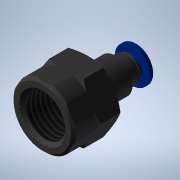
# Autodesk Inventor part: 190650 QSF-1/4-4-B
Saved by Autodesk Inventor 2021 (Build 250183000, 183)
## iProperties
Created: 2026-09-15
Part Number: 190650 QSF-1/4-4-B
Material: Generic
Catalog Web Link: www.3dfindit.com
Description: QSF-...-B-Push-in fitting
Vendor: FESTO
Document SubType Name: Modeling
Designer: psAdmin
Manufacturer: FESTO
Mass: 21 g
Surface Area: 21.8176 cm^2
Volume: 2.85568 cm^3
Density: 1 g/cm^3
Appearance: PSOLRGB-176-176-176
Category: PARTsolutions
Company: FESTO
Title: 190650 QSF-1/4-4-B
Author: Cadenas PARTsolutions
Comments: Push-in fitting
PSOL_IDENT_0: {$CADENAS_DATA/23d-libs/festo/parts/q/qsf/qsf_b.prj},179 {VTYP=3D},{NB=190650 QSF-1/4-4-B},{LINA=190
PSOL_IDENT_1: 650 QSF-1/4-4-B},{NN=QSF-...-B},{DATE=05.05.2026 15:29:25},{GEOMDATE=01.04.2025 10:00:39},{VERSION=}
PSOL_IDENT_2: ,{LINEID=40},{WBVAR=},{WBNUMERIC=}  {NB=190650 QSF-1/4-4-B},{LINA=190650 QSF-1/4-4-B},{KT=DUMMY},{TN
PSOL_IDENT_3: R=190650},{TYP=QSF-1/4-4-B},{D1=G1/4},{NENN=3.000},{D2=4},{D5=7.5},{L1=26.9},{L2=9},{SW=17},{T=14.9}
PSOL_IDENT_4: ,{CNSMASSEXACT=0.021},{D1N=13.157},{Z=9.9},{L3=20.600},{L3D1=17.600},{L3D2=9.700},{L4=7.000},{L5=7.6
PSOL_IDENT_5: 00},{GTIN=4052568042851},{REACH=Ja},{REACHSVHC=Ja},{REACHHAZSUBS=7439-92-1},{REACHSCIP=3732228b-b396
PSOL_IDENT_6: -49b9-8f0d-ee75d35d3f40},{REACHVALDATE=05.03.2025}
NB: 190650 QSF-1/4-4-B
NN: QSF-...-B
NT: Push-in fitting
NBSYN: $TNR. $TYP.
LINA: 190650 QSF-1/4-4-B
CATALOG: Festo
TNR: 190650
TYP: QSF-1/4-4-B
D1: G1/4
NENN: 3
D2: 4
D5: 7.5
L1: 26.9
L2: 9
SW: 17
T: 14.9
CNSMASSEXACT: 0.021
GTIN: 4052568042851
REACH: Yes
REACHSVHC: Yes
REACHHAZSUBS: 7439-92-1
REACHVALDATE: 05.03.2025
SUPPLIER: FESTO
ARTICLENO: 190650 QSF-1/4-4-B
BOMINFO: 190650 QSF-1/4-4-B
CREATOR: CADENAS GmbH
Autodesk Inventor part; units mm, degrees
sketch "Sketch_1" plane through (0, 0, 0) normal (1, 0, 0) x (0, 1, 0)
  line L0 (0, -26.9) -> (0, 0)
  line L1 (0, 0) -> (10.2, 0)
  line L2 (10.2, 0) -> (10.2, -20.6)
  line L3 (10.2, -20.6) -> (3.75, -20.6)
  line L4 (3.75, -20.6) -> (3.75, -23.35)
  line L5 (3.75, -23.35) -> (3.6, -23.5)
  line L6 (3.6, -23.5) -> (3.45, -23.5)
  line L7 (3.45, -23.5) -> (3.45, -23.85)
  line L8 (3.45, -23.85) -> (3.3, -24)
  line L9 (3.3, -24) -> (3.45, -24.15)
  line L10 (3.45, -24.15) -> (3.45, -24.5)
  line L11 (3.45, -24.5) -> (2.7, -24.5)
  line L12 (2.7, -24.5) -> (2.7, -25.05)
  arc A0 (2.7, -25.05) -> (3.05, -25.4) centre (3.05, -25.05) ccw
  line L13 (3.05, -25.4) -> (4.95, -25.4)
  line L14 (4.95, -25.4) -> (4.95, -26.2649)
  arc A1 (4.7847, -26.4619) -> (4.95, -26.2649) centre (4.75, -26.2649) ccw
  line L15 (4.7847, -26.4619) -> (2.3, -26.9)
  line L16 (2.3, -26.9) -> (0, -26.9)
  line L17 (0, -26.9) -> (0, 0)
  constraints: 36 end point, 4 point on circle, 2 centre point
revolve "Revolution1" add sketch "Sketch_1" angle 360 about axis through (0, 0, -26.9) along (0, 0, -1)
sketch "Sketch_2" plane through (0, 0, 0) normal (1, 0, 0) x (0, 1, 0)
  line L0 (0, -26.9) -> (0, 0)
  line L1 (0, 0) -> (6.5785, 0)
  line L2 (6.5785, 0) -> (5.7225, -0.856)
  line L3 (5.7225, -0.856) -> (5.7225, -9)
  line L4 (5.7225, -9) -> (2, -9)
  line L5 (2, -9) -> (1.5, -9.5)
  line L6 (1.5, -9.5) -> (1.5, -12)
  line L7 (1.5, -12) -> (2, -12)
  line L8 (2, -12) -> (2, -26.6)
  arc A0 (2, -26.6) -> (2.3, -26.9) centre (2.3, -26.6) ccw
  line L9 (2.3, -26.9) -> (0, -26.9)
  line L10 (0, -26.9) -> (0, 0)
  constraints: 22 end point, 2 point on circle, 1 centre point
revolve "Revolution2" cut sketch "Sketch_2" angle 360 about axis through (0, 0, -26.9) along (0, 0, -1)
thread "Thread1" size "G13.157x1.337" designation "G 1/4" standard "ISO Pipe Threads" full length
sketch "Sketch_3" plane through (0, 0, 0) normal (1, 0, 0) x (0, 1, 0)
  line L0 (0, -50) -> (0, 50)
  line L1 (8.5, 0) -> (10.2, -0.9815)
  line L2 (10.2, -0.9815) -> (10.2, -19.6185)
  line L3 (10.2, -19.6185) -> (8.5, -20.6)
  line L4 (8.5, -20.6) -> (13.5, -20.6)
  line L5 (13.5, -20.6) -> (13.5, 0)
  line L6 (13.5, 0) -> (8.5, 0)
  constraints: 14 end point
revolve "Revolution3" cut sketch "Sketch_3" angle 360 about axis through (0, 0, -50) along (0, 0, -1)
sketch "Sketch_4" plane through (0, 0, 0) normal (0, 0, 1) x (1, 0, 0)
  line L0 (-17, -17) -> (17, -17)
  line L1 (17, -17) -> (17, 17)
  line L2 (17, 17) -> (-17, 17)
  line L3 (-17, 17) -> (-17, -17)
  line L4 (-9.815, 0) -> (-4.9075, -8.5)
  line L5 (-4.9075, -8.5) -> (4.9075, -8.5)
  line L6 (4.9075, -8.5) -> (9.815, 0)
  line L7 (9.815, 0) -> (4.9075, 8.5)
  line L8 (4.9075, 8.5) -> (-4.9075, 8.5)
  line L9 (-4.9075, 8.5) -> (-9.815, 0)
  constraints: 20 end point
extrude "Extrusion1" cut sketch "Sketch_4" against normal blind 20.6
sketch "Sketch_5" plane through (0, 0, 0) normal (1, 0, 0) x (0, 1, 0)
  line L0 (0, -50) -> (0, 50)
  line L1 (8.0929, 0) -> (8.8, -0.7071)
  line L2 (8.8, -0.7071) -> (8.8, -6.1917)
  line L3 (8.8, -6.1917) -> (10.2, -7)
  line L4 (10.2, -7) -> (18.8, -7)
  line L5 (18.8, -7) -> (18.8, 0)
  line L6 (18.8, 0) -> (8.0929, 0)
  constraints: 14 end point
revolve "Revolution4" cut sketch "Sketch_5" angle 360 about axis through (0, 0, -50) along (0, 0, -1)
sketch "Sketch_6" plane through (0, 0, 0) normal (1, 0, 0) x (0, 1, 0)
  line L0 (0, -50) -> (0, 50)
  line L1 (14.85, -9.3338) -> (8.5, -13)
  line L2 (8.5, -13) -> (4.85, -13)
  line L3 (4.85, -13) -> (4.85, -20.6)
  line L4 (4.85, -20.6) -> (14.85, -20.6)
  line L5 (14.85, -20.6) -> (14.85, -9.3338)
  constraints: 12 end point
revolve "Revolution5" cut sketch "Sketch_6" angle 360 about axis through (0, 0, -50) along (0, 0, -1)
ref_plane "ANBAU_STD_XY" through (0, 0, 0) normal (0, 0, -1) x (1, 0, 0)
ref_plane "ANBAU_STD_YZ" through (0, 0, 0) normal (1, 0, 0) x (0, -1, 0)
ref_plane "ANBAU_STD_ZX" through (0, 0, 0) normal (0, -1, 0) x (0, 0, -1)
body "Solid1"
